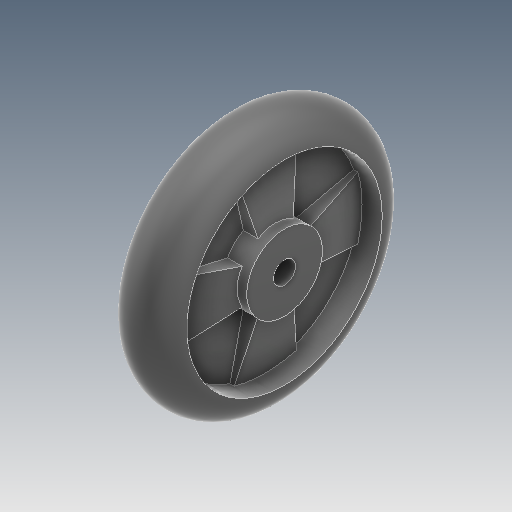
# Autodesk Inventor part: Llanta
Saved by Autodesk Inventor 2021 (Build 250183000, 183)
## iProperties
Created: 2024-03-17
Part Number: Llanta
Material: Acetal Resin, Black
Document SubType Name: Modeling
Designer: Martin
Density: 1.425 g/cm^3
Appearance: Smooth - Black
Author: Martin
Autodesk Inventor part; units mm, degrees
ref_plane "YZ Plane" through (0, 0, 0) normal (1, 0, 0) x (0, 1, 0)
sketch "Sketch1" plane through (0, 0, 0) normal (0, 1, 0) x (-1, 0, 0)
  line L0 (-17, 0) -> (17, 0)
  line L1 (17, 0) -> (17, -75)
  line L2 (17, -75) -> (-17, -75)
  line L3 (-17, -58) -> (-17, 0)
  arc A0 (-17, -58) -> (17, -58) centre (0, -58) ccw
  line L4 (23.8, 0) -> (-23.8, 0) projected
  point P0 (0, 0)
  point P1 (0, 0)
  dimension "d0" = 34
  dimension "d1" = 75
  dimension "d2" = 34
  constraints: 8 end point, 2 parallel, 2 point on circle, 2 tangent, 1 centre point, 1 horizontal, 1 midpoint, 1 perpendicular, 1 point on line
  measures "d0" distance of L1.end L2.end
  measures "d1" distance of L0.end L1.end
  measures "d2" diameter of A0
revolve "Revolution1" add sketch "Sketch1" angle 360 about axis through (-10, 0, 0) along (1, 0, 0) contours L0 L1 A0 L3
sketch "Sketch2" plane through (17, 0, 0) normal (1, 0, 0) x (0, 0, -1)
  circle A0 centre (0, 0) radius 58 projected
  circle A1 centre (0, 0) radius 22.5
  dimension "d4" = 45
  constraints: 1 centre point, 1 coincident
  measures "d4" diameter of A1
extrude "Extrusion1" cut sketch "Sketch2" against normal blind 14
sketch "Sketch3" plane through (17, 0, 0) normal (1, 0, 0) x (0, 0, -1)
  circle A0 centre (0, 0) radius 6.5
  dimension "d7" = 13
  constraints: 1 centre point, 1 coincident
  measures "d7" diameter of A0
extrude "Extrusion2" cut sketch "Sketch3" against normal blind 20
ref_plane "Work Plane1" through (0, 0, 0) normal (-0.9848, 0, -0.1736) x (0, 1, 0)
ref_plane "Work Plane2" through (14.7721, 0, 2.6047) normal (-0.9848, 0, -0.1736) x (0, 1, 0)
sketch "Sketch6" plane through (3, 0, 0) normal (1, 0, 0) x (0, 0, -1)
  circle A0 centre (0, 0) radius 58 projected
  circle A1 centre (0, 0) radius 22.5 projected
  line L0 (-54.9704, -18.5) -> (-54.9704, 18.5)
  line L1 (-19.8997, -10.5) -> (-19.8997, 10.5)
  circle A2 centre (0, 0) radius 22.5 projected
  circle A3 centre (0, 0) radius 58 projected
  line L2 (-19.8997, 10.5) -> (-54.9704, 18.5)
  line L3 (-19.8997, -10.5) -> (-54.9704, -18.5)
  dimension "d20" = 37
  dimension "d21" = 21
  constraints: 8 end point, 4 point on circle, 2 vertical
  measures "d20" distance of L0.start L0.end
  measures "d21" distance of L1.start L1.end
extrude "Extrusion4" add sketch "Sketch6" along normal up to surface contours L0 A0 | L2 A1 L3 L0 surface through (14.7721, 0, 2.6047) normal (-0.9848, 0, -0.1736)
pattern_circular "Circular Pattern1" count 4 over 360 about axis through (-10, 0, 0) along (1, 0, 0) of "Extrusion4"
mirror "Mirror1" about plane through (0, 0, 0) normal (1, 0, 0) of "Extrusion1", "Extrusion2", "Extrusion4", "Circular Pattern1"
ref_plane "Work Plane3" through (0, 0, 0) normal (1, 0, 0) x (0, 1, 0)
body "Solid1"
